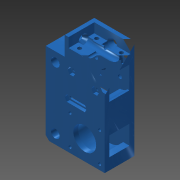
# Autodesk Inventor part: YMotorBlockLeft
Saved by Autodesk Inventor 2015 (Build 190159000, 159)
## iProperties
Created: 2014-08-14
Part Number: YMotorBlockLeft
Material: ABS Plastic
Document SubType Name: Modeling
Designer: Jack
Density: 1.06 g/cm^3
Appearance: Cyan
Author: Jack
Autodesk Inventor part; units mm, degrees
ref_plane "YZ Plane" through (0, 0, 0) normal (1, 0, 0) x (0, 1, 0)
ref_plane "XZ Plane" through (0, 0, 0) normal (0, 1, 0) x (-1, 0, 0)
ref_plane "XY Plane" through (0, 0, 0) normal (0, 0, 1) x (1, 0, 0)
sketch "Sketch1" plane through (0, 0, 0) normal (0, 1, 0) x (-1, 0, 0)
  line L0 (0, 0) -> (0, -105)
  line L1 (42, 0) -> (0, 0)
  line L2 (0, -105) -> (62, -105)
  line L3 (42, 0) -> (42, -20)
  line L4 (42, -20) -> (62, -20)
  line L5 (62, -20) -> (62, -105)
  dimension "d7" = 105
  dimension "d12" = 62
  dimension "d13" = 20
  dimension "d14" = 20
  constraints: 12 end point, 3 vertical, 2 perpendicular, 1 horizontal, 1 vertical alignment
  measures "d7" distance of L0.start L0.end
  measures "d12" distance of L0.end L2.end
  measures "d13" distance of L1.start L3.end
  measures "d14" distance of L3.end L4.end
extrude "BaseSurface" add sketch "Sketch1" along normal blind 5
sketch "Sketch2" plane through (0, 5, 0) normal (0, 1, 0) x (1, 0, 0)
  line L0 (0, 0) -> (0, 105) projected
  line L1 (0, 105) -> (-62, 105) projected
  line L2 (-62, 105) -> (-62, 20) projected
  line L3 (-62, 20) -> (-42, 20) projected
  line L4 (-42, 20) -> (-42, 0) projected
  line L5 (-42, 0) -> (0, 0) projected
  line L6 (-62, 85) -> (-44.3238, 85)
  line L7 (-6.5778, 93) -> (0, 93)
  line L8 (-8.0385, 73) -> (0, 73)
  line L9 (-10, 71.0385) -> (-10, 46)
  arc A0 (-2, 42.5498) -> (-10, 46) centre (-10, 35) ccw
  line L10 (-2, 42.5498) -> (0, 42.5498)
  arc A1 (-10, 71.0385) -> (-8.0385, 73) centre (-21, 84) ccw
  arc A2 (-6.5778, 93) -> (-36.8602, 90.12) centre (-21, 84) ccw
  arc A3 (-46, 30) -> (-35, 19) centre (-35, 30) ccw
  line L11 (-35, 19) -> (0, 19)
  line L12 (-50, 35) -> (-62, 35)
  line L13 (-46, 30) -> (-46, 31)
  arc A4 (-46, 31) -> (-50, 35) centre (-50, 31) ccw
  arc A5 (-44.3238, 85) -> (-36.8602, 90.12) centre (-44.3238, 93) ccw
  point P0 (-37.9706, 85)
  point P1 (-46, 35)
  dimension "d17" = 21
  dimension "d18" = 21
  dimension "d19" = 20
  dimension "d20" = 12
  dimension "d21" = 32
  dimension "d22" = 10
  dimension "d24" = 35
  dimension "d25" = 10
  dimension "d26" = 2
  dimension "d27" = 17
  dimension "d28" = 17
  dimension "d29" = 11
  dimension "d31" = 30
  dimension "d32" = 27
  dimension "d33" = 15
  dimension "d34" = 11
  dimension "d47" = 4
  dimension "d48" = 8
  constraints: 16 end point, 13 point on circle, 9 point on line, 6 centre point, 6 perpendicular, 6 tangent, 1 horizontal, 1 vertical
  measures "d17" distance from line of L0 A1.centre
  measures "d18" distance from line of L1 A1.centre
  measures "d19" distance between parallel lines of L1 L6
  measures "d20" distance between parallel lines of L1 L7
  measures "d21" distance between parallel lines of L1 L8
  measures "d22" distance between parallel lines of L0 L9
  measures "d24" distance from line of L5 A0.centre
  measures "d25" distance from line of L0 A0.centre
  measures "d26" distance of L10.start L10.end
  measures "d27" radius of A1
  measures "d28" radius of A2
  measures "d29" radius of A0
  measures "d31" distance from line of L5 A3.centre
  measures "d32" distance from line of L2 A3.centre
  measures "d33" distance between parallel lines of L3 L12
  measures "d34" radius of A3
  measures "d47" radius of A4
  measures "d48" radius of A5
extrude "InternalFill" add sketch "Sketch2" along normal blind 21 contours L5 L4 L3 L2 L12 A4 L13 A3 L11 L0 | L10 A0 L9 A1 L8 L0 | L7 A2 A5 L6 L2 L1 L0
sketch "Sketch5" plane through (0, 26, 0) normal (0, 1, 0) x (1, 0, 0)
  line L0 (-42, 20) -> (-42, 0) projected
  line L1 (-42, 0) -> (0, 0) projected
  line L2 (-38, 0) -> (-38, 10)
  line L3 (-38, 10) -> (0, 10)
  line L4 (0, 0) -> (0, 105) projected
  dimension "d43" = 4
  dimension "d44" = 10
  constraints: 4 end point, 2 point on line, 1 perpendicular, 1 vertical
  measures "d43" distance between parallel lines of L0 L2
  measures "d44" distance between parallel lines of L1 L3
extrude "YRodNotch" cut sketch "Sketch5" against normal up to surface (26 mm away)
sketch "Sketch6" plane through (0, 26, 0) normal (0, 1, 0) x (1, 0, 0)
  line L0 (-38, 0) -> (-38, 10) projected
  line L1 (-38, 10) -> (0, 10) projected
  line L2 (-62, 20) -> (-42, 20) projected
  line L3 (-42, 20) -> (-42, 0) projected
  line L4 (-42, 0) -> (-38, 0) projected
  arc A0 (-10, 71.0385) -> (-8.0385, 73) centre (-21, 84) ccw projected
  line L5 (-10, 71.0385) -> (-10, 46) projected
  arc A1 (-2, 42.5498) -> (-10, 46) centre (-10, 35) ccw projected
  line L6 (-2, 42.5498) -> (0, 42.5498) projected
  line L7 (0, 42.5498) -> (0, 73) projected
  line L8 (0, 73) -> (-8.0385, 73) projected
  line L9 (0, 105) -> (-62, 105) projected
  line L10 (-62, 105) -> (-62, 85) projected
  line L11 (-62, 85) -> (-44.3238, 85) projected
  arc A2 (-44.3238, 85) -> (-36.8602, 90.12) centre (-44.3238, 93) ccw projected
  arc A3 (-6.5778, 93) -> (-36.8602, 90.12) centre (-21, 84) ccw projected
  line L12 (-6.5778, 93) -> (0, 93) projected
  line L13 (0, 93) -> (0, 105) projected
  line L14 (-62, 20) -> (-62, 105)
  line L15 (-62, 105) -> (-62, 20) projected
  line L16 (-62, 105) -> (0, 105)
  line L17 (0, 105) -> (0, 10)
  line L18 (0, 10) -> (-38, 10)
  line L19 (0, 10) -> (0, 19) projected
  line L20 (-38, 0) -> (0, 0)
  line L21 (0, 0) -> (0, 10)
  point P0 (-62, 35)
  constraints: 12 end point, 3 collinear, 1 horizontal, 1 perpendicular, 1 vertical
extrude "TopSurface" add sketch "Sketch6" along normal blind 5
sketch "Sketch3" plane through (0, 0, 0) normal (0, -1, 0) x (1, 0, 0)
  arc A0 (-36.8602, -90.12) -> (-6.5778, -93) centre (-21, -84) ccw projected
  arc A1 (-36.8602, -90.12) -> (-6.5778, -93) centre (-21, -84) ccw projected
  circle A2 centre (-21, -84) radius 12
  dimension "d37" = 24
  constraints: 1 centre point, 1 coincident
  measures "d37" diameter of A2
extrude "MotorBulgeRecess" cut sketch "Sketch3" against normal up to surface (5 mm away)
sketch "Sketch7" plane through (0, 31, 0) normal (0, 1, 0) x (1, 0, 0)
  line L0 (0, 0) -> (0, 105) projected
  line L1 (0, 105) -> (-62, 105) projected
  point P0 (0, 10)
  point P1 (-5.5, 68.5)
  point P2 (-5.5, 99.5)
  point P3 (-36.5, 99.5)
  point P4 (-36.5, 68.5)
  dimension "d51" = 31
  dimension "d52" = 31
  dimension "d53" = 5.5
  dimension "d54" = 5.5
  constraints: 2 horizontal alignment, 2 vertical alignment
  measures "d51" distance of point (-36.5, 99.5) point (-36.5, 68.5)
  measures "d52" distance of point (-5.5, 68.5) point (-36.5, 68.5)
  measures "d53" distance from line of L0 point (-5.5, 99.5)
  measures "d54" distance from line of L1 point (-5.5, 99.5)
hole "MotorMountHoles" at (-5.5, 31, -68.5) at (-5.5, 31, -99.5) at (-36.5, 31, -99.5) at (-36.5, 31, -68.5) direction (0, -1, 0) diameter 3 end through all counterbore diameter 6 counterbore depth 28
sketch "Sketch8" plane through (0, 31, 0) normal (0, 1, 0) x (1, 0, 0)
  arc A0 (-2, 42.5498) -> (-10, 46) centre (-10, 35) ccw projected
  arc A1 (-46, 30) -> (-35, 19) centre (-35, 30) ccw projected
  arc A2 (-46, 30) -> (-35, 19) centre (-35, 30) ccw projected
hole "IdlerBearingHoles" at (-35, 31, -30) at (-10, 31, -35) direction (0, -1, 0) diameter 4 end through all counterbore diameter 7 counterbore depth 4
sketch "Sketch9" plane through (0, 0, 0) normal (0, -1, 0) x (1, 0, 0)
  circle A0 centre (-35, -30) radius 2 projected
  circle A1 centre (-10, -35) radius 2 projected
  line L0 (-12.0207, -38.5) -> (-14.0415, -35)
  line L1 (-14.0415, -35) -> (-12.0207, -31.5)
  line L2 (-12.0207, -31.5) -> (-7.9793, -31.5)
  line L3 (-7.9793, -31.5) -> (-5.9585, -35)
  line L4 (-5.9585, -35) -> (-7.9793, -38.5)
  line L5 (-7.9793, -38.5) -> (-12.0207, -38.5)
  line L6 (-32.9793, -33.5) -> (-37.0207, -33.5)
  line L7 (-37.0207, -33.5) -> (-39.0415, -30)
  line L8 (-39.0415, -30) -> (-37.0207, -26.5)
  line L9 (-37.0207, -26.5) -> (-32.9793, -26.5)
  line L10 (-32.9793, -26.5) -> (-30.9585, -30)
  line L11 (-30.9585, -30) -> (-32.9793, -33.5)
  point P0 (0, 0)
  point P1 (-10, -35)
  point P2 (-35, -30)
  dimension "d69" = 7
  constraints: 24 end point, 2 coincident, 2 horizontal, 1 equal length, 26 other
  measures "d69" distance between parallel lines of L4 L1
extrude "IdlerBearingNutTrap" cut sketch "Sketch9" against normal blind 3.2
sketch "Sketch10" plane through (0, 31, 0) normal (0, 1, 0) x (1, 0, 0)
  line L0 (0, 105) -> (-62, 105) projected
  line L1 (-62, 105) -> (-62, 20) projected
  line L2 (-23, 56.5) -> (-38, 56.5) construction
  line L3 (-23, 58.5) -> (-38, 58.5)
  line L4 (-38, 54.5) -> (-23, 54.5)
  arc A0 (-23, 54.5) -> (-23, 58.5) centre (-23, 56.5) ccw
  arc A1 (-38, 58.5) -> (-38, 54.5) centre (-38, 56.5) ccw
  point P0 (-30.5, 56.5)
  dimension "d72" = 15
  dimension "d73" = 4
  dimension "d74" = 48.5
  dimension "d75" = 24
  constraints: 8 end point, 4 point on circle, 4 tangent, 2 centre point, 1 horizontal, 1 midpoint, 1 parallel
  measures "d72" distance of L2.start L2.end
  measures "d73" diameter of A1
  measures "d74" distance from line of L0 L2.end
  measures "d75" distance from line of L1 L2.end
extrude "TensionerBearingSlot" cut sketch "Sketch10" against normal up to surface (31 mm away)
sketch "Sketch11" plane through (0, 31, 0) normal (0, 1, 0) x (1, 0, 0)
  line L0 (-38, 58.5) -> (-23, 58.5) projected
  arc A0 (-23, 54.5) -> (-23, 58.5) centre (-23, 56.5) ccw projected
  line L1 (-23, 54.5) -> (-38, 54.5) projected
  arc A1 (-38, 58.5) -> (-38, 54.5) centre (-38, 56.5) ccw projected
  line L2 (-23, 56.5) -> (-38, 56.5) construction
  line L3 (-23, 60) -> (-38, 60)
  line L4 (-38, 53) -> (-23, 53)
  arc A2 (-23, 53) -> (-23, 60) centre (-23, 56.5) ccw
  arc A3 (-38, 60) -> (-38, 53) centre (-38, 56.5) ccw
  point P0 (-30.5, 56.5)
  dimension "d78" = 7
  constraints: 8 end point, 4 point on circle, 4 tangent, 2 centre point, 1 horizontal, 1 midpoint, 1 parallel
  measures "d78" diameter of A3
extrude "TensionerBearingHeadSlot" cut sketch "Sketch11" against normal blind 4
sketch "Sketch12" plane through (0, 0, 0) normal (0, -1, 0) x (1, 0, 0)
  arc A0 (-38, -54.5) -> (-38, -58.5) centre (-38, -56.5) ccw projected
  arc A1 (-23, -58.5) -> (-23, -54.5) centre (-23, -56.5) ccw projected
  line L0 (-18.9585, -56.5) -> (-20.9793, -60)
  line L1 (-20.9793, -60) -> (-25.0207, -60)
  line L2 (-25.0207, -60) -> (-27.0415, -56.5)
  line L3 (-27.0415, -56.5) -> (-25.0207, -53)
  line L4 (-25.0207, -53) -> (-20.9793, -53)
  line L5 (-20.9793, -53) -> (-18.9585, -56.5)
  line L6 (-42.0415, -56.5) -> (-40.0207, -53)
  line L7 (-40.0207, -53) -> (-35.9793, -53)
  line L8 (-35.9793, -53) -> (-33.9585, -56.5)
  line L9 (-33.9585, -56.5) -> (-35.9793, -60)
  line L10 (-35.9793, -60) -> (-40.0207, -60)
  line L11 (-40.0207, -60) -> (-42.0415, -56.5)
  line L12 (-35.9793, -53) -> (-25.0207, -53)
  line L13 (-23, -53) -> (-38, -53) projected
  line L14 (-25.0207, -60) -> (-35.9793, -60)
  line L15 (-38, -60) -> (-23, -60) projected
  point P0 (0, 0)
  point P1 (-23, -56.5)
  point P2 (-38, -56.5)
  dimension "d81" = 7
  constraints: 28 end point, 2 coincident, 2 collinear, 2 horizontal, 1 horizontal alignment, 26 other
  measures "d81" distance between parallel lines of L1 L4
extrude "TensionerBearingNutSlot" cut sketch "Sketch12" against normal blind 3.2
sketch "Sketch13" plane through (0, 0, 0) normal (0, -1, 0) x (1, 0, 0)
  line L0 (-62, -20) -> (-42, -20) projected
  line L1 (-62, -105) -> (-62, -20) projected
  line L2 (0, -105) -> (-62, -105) projected
  point P0 (0, 0)
  point P1 (-52, -30)
  point P2 (-52, -95)
  dimension "d84" = 10
  dimension "d85" = 10
  dimension "d86" = 10
  constraints: 1 vertical alignment
  measures "d84" distance from line of L1 point (-52, -30)
  measures "d85" distance from line of L0 point (-52, -30)
  measures "d86" distance from line of L2 point (-52, -95)
hole "FrameMountHolesBack" at (-52, 0, -30) at (-52, 0, -95) direction (0, 1, 0) diameter 5 end through all counterbore diameter 9 counterbore depth 29
sketch "Sketch14" plane through (0, 0, -10) normal (1, 0, 0) x (0, 0, -1)
  line L0 (-10, 31) -> (95, 31) projected
  line L1 (0, 26) -> (0, 0) projected
  circle A0 centre (0, 15.5) radius 4
  point P0 (-10, 0)
  dimension "d94" = 8
  dimension "d96" = 15.5
  constraints: 1 centre point, 1 point on line
  measures "d94" diameter of A0
  measures "d96" distance from line of L0 A0.centre
extrude "YRodHole" cut sketch "Sketch14" against normal up to surface (38 mm away)
sketch "Sketch18" plane through (-38, 19.5, -10) normal (0, 0, 1) x (1, 0, 0)
  line L0 (0, 0) -> (38, 0) projected
  line L1 (0, -8) -> (0, 0) projected
  line L2 (38, -8) -> (0, -8) projected
  line L3 (38, 0) -> (38, -8) projected
  line L4 (38, -8) -> (38, -19.5) projected
  line L5 (38, -8) -> (0, -8) projected
  line L6 (0, -8) -> (0, -19.5) projected
  line L7 (38, -11.5) -> (38, -16.5) projected
  circle A0 centre (32, 4) radius 2
  circle A1 centre (6, 4) radius 2
  circle A2 centre (6, -14) radius 2
  circle A3 centre (32, -14) radius 2
  line L8 (38, -19.5) -> (0, -19.5) projected
  line L9 (0, 0) -> (38, 0) projected
  line L10 (38, 6.5) -> (38, 0) projected
  line L11 (0, 6.5) -> (38, 6.5) projected
  line L12 (0, 6.5) -> (0, 0) projected
  dimension "d113" = 4
  dimension "d114" = 4
  dimension "d115" = 4
  dimension "d116" = 4
  dimension "d117" = 6
  dimension "d120" = 32
  dimension "d159" = 4
  dimension "d160" = 6
  constraints: 4 centre point, 2 horizontal alignment, 2 vertical alignment
  measures "d113" diameter of A0
  measures "d114" diameter of A1
  measures "d115" diameter of A2
  measures "d116" diameter of A3
  measures "d117" distance from line of L7 A3.centre
  measures "d120" distance from line of L7 A2.centre
  measures "d159" distance from line of L0 A0.centre
  measures "d160" distance from line of L2 A3.centre
extrude "YRodClampHoles" cut sketch "Sketch18" against normal up to surface (9 mm away) contours A0 | A1 | A2 | A3
sketch "Sketch19" plane through (0, 26, -19) normal (0, 0, -1) x (-1, 0, 0)
  circle A0 centre (32, -20.5) radius 2 projected
  circle A1 centre (6, -20.5) radius 2 projected
  circle A2 centre (32, -2.5) radius 2 projected
  circle A3 centre (6, -2.5) radius 2 projected
  line L0 (10.0415, -2.5) -> (8.0207, -6)
  line L1 (8.0207, -6) -> (3.9793, -6)
  line L2 (3.9793, -6) -> (1.9585, -2.5)
  line L3 (1.9585, -2.5) -> (3.9793, 1)
  line L4 (3.9793, 1) -> (8.0207, 1)
  line L5 (8.0207, 1) -> (10.0415, -2.5)
  line L6 (10.0415, -20.5) -> (8.0207, -24)
  line L7 (8.0207, -24) -> (3.9793, -24)
  line L8 (3.9793, -24) -> (1.9585, -20.5)
  line L9 (1.9585, -20.5) -> (3.9793, -17)
  line L10 (3.9793, -17) -> (8.0207, -17)
  line L11 (8.0207, -17) -> (10.0415, -20.5)
  line L12 (36.0415, -20.5) -> (34.0207, -24)
  line L13 (34.0207, -24) -> (29.9793, -24)
  line L14 (29.9793, -24) -> (27.9585, -20.5)
  line L15 (27.9585, -20.5) -> (29.9793, -17)
  line L16 (29.9793, -17) -> (34.0207, -17)
  line L17 (34.0207, -17) -> (36.0415, -20.5)
  line L18 (36.0415, -2.5) -> (34.0207, -6)
  line L19 (34.0207, -6) -> (29.9793, -6)
  line L20 (29.9793, -6) -> (27.9585, -2.5)
  line L21 (27.9585, -2.5) -> (29.9793, 1)
  line L22 (29.9793, 1) -> (34.0207, 1)
  line L23 (34.0207, 1) -> (36.0415, -2.5)
  point P0 (30.0635, -21)
  point P1 (33.9365, -21)
  point P2 (4.0635, -21)
  point P3 (7.9365, -21)
  point P4 (0, -26)
  dimension "d123" = 7
  constraints: 48 end point, 4 coincident, 4 horizontal, 3 equal length, 52 other
  measures "d123" distance between parallel lines of L19 L22
extrude "YRodClampNutTraps" cut sketch "Sketch19" along normal blind 3.2 and the other way blind 3.2 contours A0 | A1 | L0 L1 L2 L3 L4 L5 | L6 L7 L8 L9 L10 L11 | L12 L13 L14 L15 L16 L17 | L18 L19 L20 L21 L22 L23
sketch "Sketch26" plane through (-38, 0, 0) normal (1, 0, 0) x (0, 0, -1)
  arc A0 (10, 11.5) -> (10, 19.5) centre (10, 15.5) ccw projected
  circle A1 centre (10, 15.5) radius 2.5
  dimension "d161" = 5
  constraints: 1 centre point, 1 coincident
  measures "d161" diameter of A1
extrude "FrameMountHoleSideVert" cut sketch "Sketch26" against normal up to surface (4 mm away)
sketch "Sketch32" plane through (0, 26, 0) normal (0, -1, 0) x (1, 0, 0)
  line L0 (-38, 0) -> (-38, -10) projected
  line L1 (-38, -10) -> (0, -10) projected
  line L2 (0, 0) -> (0, -10) projected
  line L3 (-38, 0) -> (0, 0) projected
extrude "Extrusion27" cut sketch "Sketch32" against normal blind 1
sketch "Sketch33" plane through (-38, 19.5, -10) normal (0, 0, 1) x (1, 0, 0)
  line L0 (0, 7.5) -> (0, 0) projected
  line L1 (0, -1.5) -> (-4, -1.5) projected
  line L2 (0, -1.5) -> (0, 1.1)
  line L3 (0, 1.1) -> (-3.6, -1.5)
  line L4 (-3.6, -1.5) -> (0, -1.5)
  line L5 (0, -8) -> (0, 0) projected
  line L6 (0, -4) -> (-4, -4)
  point P0 (38, -19.5)
  dimension "d184" = 2.6
  dimension "d185" = 3.6
  constraints: 8 end point, 2 point on line, 1 collinear, 1 horizontal, 1 midpoint
  measures "d184" distance of L1.start L2.end
  measures "d185" distance from line of L2 L3.end
revolve "Revolution3" cut sketch "Sketch33" angle 360 about axis through (-38, 15.5, -10) along (-1, 0, 0)
sketch "Sketch34" plane through (-38, 10.4, -10) normal (-1, 0, 0) x (0, 0, 1)
  line L0 (0, 1.1) -> (0, 0) projected
  arc A0 (0, 9.1) -> (0, 1.1) centre (0, 5.1) ccw projected
  line L1 (0, 10.2) -> (0, 9.1) projected
  arc A1 (0, 10.2) -> (0, 0) centre (0, 5.1) ccw projected
  point P0 (10, -10.4)
extrude "Extrusion28" cut sketch "Sketch34" against normal blind 6
sketch "Sketch35" plane through (0, 27, 0) normal (0, -1, 0) x (1, 0, 0)
  line L0 (0, -10) -> (-38, -10) projected
  line L1 (0, 0) -> (0, -10) projected
  circle A0 centre (-19, -10) radius 2.5
  dimension "d189" = 5
  dimension "d190" = 19
  constraints: 1 centre point, 1 midpoint
  measures "d189" diameter of A0
  measures "d190" distance from line of L1 A0.centre
extrude "Extrusion29" cut sketch "Sketch35" against normal up to surface (4 mm away)
sketch "Sketch36" plane through (0, 19.5, -10) normal (0, 0, 1) x (1, 0, 0)
  line L0 (0, 7.5) -> (-16.5, 7.5) projected
  line L1 (-21.5, 11.5) -> (-16.5, 11.5) projected
  line L2 (-16.5, 7.5) -> (-21.5, 7.5) projected
  line L3 (-21.5, 7.5) -> (-16.5, 7.5) projected
  line L4 (-13.9, 7.5) -> (-16.5, 11.1)
  line L5 (-16.5, 11.1) -> (-16.5, 7.5)
  line L6 (-16.5, 7.5) -> (-21.5, 7.5) projected
  line L7 (-16.5, 7.5) -> (-13.9, 7.5)
  line L8 (0, 11.5) -> (-62, 11.5) projected
  line L9 (-19, 11.5) -> (-19, 7.5)
  point P0 (0, -19.5)
  dimension "d193" = 2.6
  dimension "d194" = 3.6
  constraints: 8 end point, 2 point on line, 1 collinear, 1 midpoint, 1 perpendicular, 1 vertical
  measures "d193" distance of L2.start L4.start
  measures "d194" distance of L4.end L2.start
revolve "Revolution4" cut sketch "Sketch36" angle 360 about axis through (-19, 31, -10) along (0, -1, 0)
sketch "Sketch37" plane through (0, 27, 0) normal (0, 1, 0) x (1, 0, 0)
  line L0 (-13.9, 10) -> (-24.1, 10) projected
  arc A0 (-13.9, 10) -> (-24.1, 10) centre (-19, 10) ccw projected
  point P0 (0, 0)
extrude "Extrusion30" cut sketch "Sketch37" against normal blind 6
sketch "Sketch38" plane through (0, 0, 0) normal (0, -1, 0) x (1, 0, 0)
  circle A0 centre (-19, -10) radius 2.5 projected
  circle A1 centre (-19, -10) radius 1.8
  point P0 (0, 0)
  dimension "d198" = 3.6
  constraints: 1 centre point, 1 coincident
  measures "d198" diameter of A1
extrude "Extrusion31" cut sketch "Sketch38" against normal up to surface (31 mm away) contours A1
body "Solid1"
